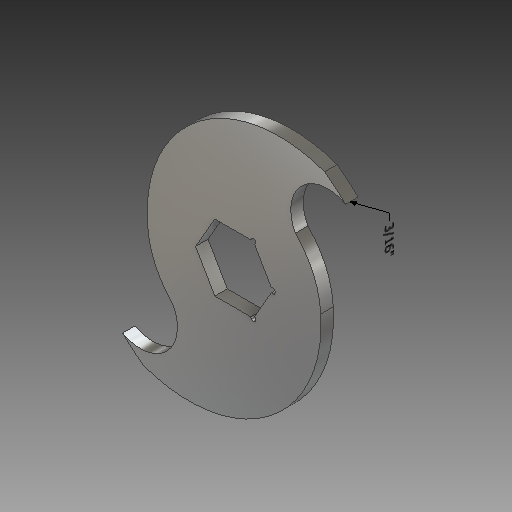
# Autodesk Inventor part: 3-16inch_Knife3_Piece1
Saved by Autodesk Inventor 2018 (Build 220112000, 112)
## iProperties
Created: 2018-01-21
Part Number: 3-16inch_Knife3_Piece1
Material: Generic
Document SubType Name: Modeling
Designer: Olivier
Density: 1 g/cm^3
Appearance: Default
Mass: 22.6409 g
Surface Area: 115.891 cm^2
Volume: 22.6409 cm^3
Author: Olivier
Autodesk Inventor part; units mm, degrees
ref_plane "YZ Plane" through (0, 0, 0) normal (1, 0, 0) x (0, 1, 0)
ref_plane "XZ Plane" through (0, 0, 0) normal (0, 1, 0) x (-1, 0, 0)
ref_plane "XY Plane" through (0, 0, 0) normal (0, 0, 1) x (1, 0, 0)
sketch "Sketch1" plane through (0, 0, 0) normal (0, 0, 1) x (1, 0, 0)
  arc A0 (-107.9651, -1.5164) -> (-98.3345, -23.3345) centre (-75, 0) ccw
  arc A1 (-40.5736, 49.1408) -> (-107.9651, -1.5164) centre (-57.8736, 2.0002) ccw
  arc A2 (-32.5736, 42.4264) -> (-40.5736, 49.1408) centre (-75, 0) ccw
  arc A3 (-32.5736, 42.4264) -> (-51.6655, 23.3345) centre (-39.3901, 30.151) ccw
  arc A4 (-42.0349, 1.5164) -> (-51.6655, 23.3345) centre (-75, 0) ccw
  arc A5 (-109.4264, -49.1408) -> (-42.0349, 1.5164) centre (-92.1264, -2.0002) ccw
  arc A6 (-117.4264, -42.4264) -> (-109.4264, -49.1408) centre (-75, 0) ccw
  arc A7 (-117.4264, -42.4264) -> (-98.3345, -23.3345) centre (-110.6099, -30.151) ccw
  arc A8 (-32.5736, 42.4264) -> (-40.5736, 49.1408) centre (-75, 0) ccw
  arc A9 (-40.5736, 49.1408) -> (-107.9651, -1.5164) centre (-57.8736, 2.0002) ccw
  arc A10 (-107.9651, -1.5164) -> (-98.3345, -23.3345) centre (-75, 0) ccw
  arc A11 (-117.4264, -42.4264) -> (-98.3345, -23.3345) centre (-110.6099, -30.151) ccw
  arc A12 (-117.4264, -42.4264) -> (-109.4264, -49.1408) centre (-75, 0) ccw
  arc A13 (-109.4264, -49.1408) -> (-42.0349, 1.5164) centre (-92.1264, -2.0002) ccw
  arc A14 (-42.0349, 1.5164) -> (-51.6655, 23.3345) centre (-75, 0) ccw
  arc A15 (-32.5736, 42.4264) -> (-51.6655, 23.3345) centre (-39.3901, 30.151) ccw
  line L0 (-82.3323, -12.7) -> (-89.6647, 0)
  line L1 (-89.6647, 0) -> (-82.3323, 12.7)
  line L2 (-82.3323, 12.7) -> (-68.6677, 12.7)
  arc A16 (-67.1677, 11.834) -> (-68.6677, 12.7) centre (-67.6677, 12.7) ccw
  line L3 (-67.1677, 11.834) -> (-60.8353, 0.866)
  arc A17 (-60.8353, -0.866) -> (-60.8353, 0.866) centre (-60.3353, 0) ccw
  line L4 (-60.8353, -0.866) -> (-67.1677, -11.834)
  arc A18 (-68.6677, -12.7) -> (-67.1677, -11.834) centre (-67.6677, -12.7) ccw
  line L5 (-68.6677, -12.7) -> (-82.3323, -12.7)
  point P0 (0, 0)
  constraints: 38 point on circle, 19 centre point, 12 end point
extrude "Extrusion1" add sketch "Sketch1" along normal blind 4.7625
body "Solid1"
